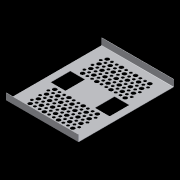
# Autodesk Inventor part: Belly Pan
Saved by Autodesk Inventor 2014 SP1 (Build 180222100, 222)
## iProperties
Created: 2013-11-29
Part Number: Belly Pan
Material: Aluminum 6061
Document SubType Name: Sheet Metal
Designer: Rauhul Varma
Mass: 3080.17 g
Surface Area: 7653.53 cm^2
Volume: 1136.59 cm^3
Density: 2.71 g/cm^3
Sheet Metal Rule: Default
Appearance: Aluminum - Flat
Flat Pattern Width: 55.88 cm
Flat Pattern Length: 83.9863 cm
Flat Pattern Area: 4693.16 cm^2
Sheet Metal Width: 22.000 in
Sheet Metal Length: 33.065 in
Sheet Metal Area: 727.441 in^2
Author: Rauhul Varma
Autodesk Inventor part; units mm, degrees
ref_plane "YZ Plane" through (0, 0, 0) normal (1, 0, 0) x (0, 1, 0)
ref_plane "XZ Plane" through (0, 0, 0) normal (0, 1, 0) x (-1, 0, 0)
sketch "Sketch2" plane through (0, 0, 0) normal (0, 1, 0) x (-1, 0, 0)
  line L0 (0, 0) -> (558.8, 0)
  line L1 (558.8, 0) -> (558.8, 736.6)
  line L2 (558.8, 736.6) -> (0, 736.6)
  line L3 (0, 736.6) -> (0, 0)
  line L4 (50.8, 736.6) -> (50.8, 0)
  line L5 (508, 736.6) -> (508, 0)
  line L6 (50.8, 698.5) -> (508, 698.5)
  line L7 (508, 38.1) -> (50.8, 38.1)
  line L8 (0, 368.3) -> (558.8, 368.3)
  line L9 (50.8, 444.5) -> (165.1, 444.5)
  line L10 (165.1, 444.5) -> (165.1, 292.1)
  line L11 (165.1, 292.1) -> (50.8, 292.1)
  line L12 (508, 292.1) -> (393.7, 292.1)
  line L13 (393.7, 292.1) -> (393.7, 444.5)
  line L14 (393.7, 444.5) -> (508, 444.5)
  line L15 (63.5, 698.5) -> (63.5, 457.2)
  line L16 (63.5, 457.2) -> (177.8, 457.2)
  line L17 (177.8, 457.2) -> (177.8, 279.4)
  line L18 (177.8, 279.4) -> (63.5, 279.4)
  line L19 (63.5, 279.4) -> (63.5, 38.1)
  line L20 (495.3, 698.5) -> (495.3, 457.2)
  line L21 (495.3, 457.2) -> (381, 457.2)
  line L22 (381, 457.2) -> (381, 279.4)
  line L23 (381, 279.4) -> (495.3, 279.4)
  line L24 (495.3, 279.4) -> (495.3, 38.1)
  circle A0 centre (85.725, 676.275) radius 22.225
  circle A1 centre (85.725, 598.805) radius 22.225
  circle A2 centre (85.725, 521.335) radius 22.225
  circle A3 centre (163.195, 676.275) radius 22.225
  circle A4 centre (163.195, 598.805) radius 22.225
  circle A5 centre (163.195, 521.335) radius 22.225
  circle A6 centre (240.665, 676.275) radius 22.225
  circle A7 centre (240.665, 598.805) radius 22.225
  circle A8 centre (240.665, 521.335) radius 22.225
  circle A9 centre (318.135, 676.275) radius 22.225
  circle A10 centre (318.135, 598.805) radius 22.225
  circle A11 centre (318.135, 521.335) radius 22.225
  circle A12 centre (395.605, 676.275) radius 22.225
  circle A13 centre (395.605, 598.805) radius 22.225
  circle A14 centre (395.605, 521.335) radius 22.225
  circle A15 centre (473.075, 676.275) radius 22.225
  circle A16 centre (473.075, 598.805) radius 22.225
  circle A17 centre (473.075, 521.335) radius 22.225
  circle A18 centre (85.725, 60.325) radius 22.225
  circle A19 centre (85.725, 137.795) radius 22.225
  circle A20 centre (85.725, 215.265) radius 22.225
  circle A21 centre (163.195, 60.325) radius 22.225
  circle A22 centre (163.195, 137.795) radius 22.225
  circle A23 centre (163.195, 215.265) radius 22.225
  circle A24 centre (240.665, 60.325) radius 22.225
  circle A25 centre (240.665, 137.795) radius 22.225
  circle A26 centre (240.665, 215.265) radius 22.225
  circle A27 centre (318.135, 60.325) radius 22.225
  circle A28 centre (318.135, 137.795) radius 22.225
  circle A29 centre (318.135, 215.265) radius 22.225
  circle A30 centre (395.605, 60.325) radius 22.225
  circle A31 centre (395.605, 137.795) radius 22.225
  circle A32 centre (395.605, 215.265) radius 22.225
  circle A33 centre (473.075, 60.325) radius 22.225
  circle A34 centre (473.075, 137.795) radius 22.225
  circle A35 centre (473.075, 215.265) radius 22.225
  line L25 (85.725, 676.275) -> (163.195, 598.805) construction
  line L26 (163.195, 676.275) -> (85.725, 598.805) construction
  circle A36 centre (124.46, 637.54) radius 17.4625
  circle A37 centre (124.46, 560.07) radius 17.4625
  circle A38 centre (201.93, 637.54) radius 17.4625
  circle A39 centre (201.93, 560.07) radius 17.4625
  circle A40 centre (279.4, 637.54) radius 17.4625
  circle A41 centre (279.4, 560.07) radius 17.4625
  circle A42 centre (356.87, 637.54) radius 17.4625
  circle A43 centre (356.87, 560.07) radius 17.4625
  circle A44 centre (434.34, 637.54) radius 17.4625
  circle A45 centre (434.34, 560.07) radius 17.4625
  line L27 (85.725, 60.325) -> (163.195, 137.795) construction
  line L28 (163.195, 60.325) -> (85.725, 137.795) construction
  circle A46 centre (124.46, 99.06) radius 17.4625
  circle A47 centre (124.46, 176.53) radius 17.4625
  circle A48 centre (201.93, 99.06) radius 17.4625
  circle A49 centre (201.93, 176.53) radius 17.4625
  circle A50 centre (279.4, 99.06) radius 17.4625
  circle A51 centre (279.4, 176.53) radius 17.4625
  circle A52 centre (356.87, 99.06) radius 17.4625
  circle A53 centre (356.87, 176.53) radius 17.4625
  circle A54 centre (434.34, 99.06) radius 17.4625
  circle A55 centre (434.34, 176.53) radius 17.4625
  dimension "d2" = 558.8
  dimension "d3" = 736.6
  dimension "d25" = 50.8
  dimension "d26" = 50.8
  dimension "d27" = 38.1
  dimension "d28" = 38.1
  dimension "d29" = 114.3
  dimension "d30" = 114.3
  dimension "d31" = 152.4
  dimension "d32" = 152.4
  dimension "d33" = 12.7
  dimension "d34" = 12.7
  dimension "d35" = 12.7
  dimension "d36" = 12.7
  dimension "d37" = 12.7
  dimension "d38" = 12.7
  dimension "d39" = 12.7
  dimension "d40" = 12.7
  dimension "d41" = 12.7
  dimension "d42" = 12.7
  dimension "d43" = 44.45
  dimension "d46" = 77.47
  dimension "d49" = 77.47
  dimension "d52" = 44.45
  dimension "d55" = 77.47
  dimension "d58" = 77.47
  dimension "d61" = 34.925
  dimension "d64" = 77.47
  dimension "d67" = 77.47
  dimension "d70" = 34.925
  dimension "d73" = 77.47
  dimension "d76" = 77.47
  constraints: 58 end point, 56 centre point, 16 point on line, 14 perpendicular, 8 parallel, 5 horizontal, 4 midpoint, 4 tangent, 4 vertical, 1 collinear, 106 other
  measures "d2" distance of L2.end L1.end
  measures "d3" distance of L1.end L0.end
  measures "d25" distance between parallel lines of L4 L3
  measures "d26" distance between parallel lines of L1 L5
  measures "d27" distance between parallel lines of L6 L2
  measures "d28" distance between parallel lines of L7 L0
  measures "d29" distance of L13.end L14.end
  measures "d30" distance of L9.start L9.end
  measures "d31" distance between parallel lines of L11 L9
  measures "d32" distance between parallel lines of L12 L14
  measures "d33" distance between parallel lines of L15 L4
  measures "d34" distance between parallel lines of L16 L9
  measures "d35" distance between parallel lines of L17 L10
  measures "d36" distance between parallel lines of L11 L18
  measures "d37" distance between parallel lines of L4 L19
  measures "d38" distance between parallel lines of L5 L20
  measures "d39" distance between parallel lines of L21 L14
  measures "d40" distance between parallel lines of L22 L13
  measures "d41" distance between parallel lines of L12 L23
  measures "d42" distance between parallel lines of L5 L24
  measures "d43" diameter of A0
  measures "d46" distance of L25.start L26.end
  measures "d49" distance of L25.start L26.start
  measures "d52" diameter of A18
  measures "d55" distance of L27.start L28.end
  measures "d58" distance of L27.start L28.start
  measures "d61" diameter of A36
  measures "d64" distance of A36.centre A37.centre
  measures "d67" distance of A36.centre A38.centre
  measures "d70" diameter of A46
  measures "d73" distance of A46.centre A47.centre
  measures "d76" distance of A46.centre A48.centre
extrude "Plate1" add sketch "Sketch2" along normal blind 3.175 contours L3 L8 L4 L0 | L4 L7 L5 L0 | L3 L2 L4 L8 | L5 L8 L1 L0 | L4 L11 L10 L8 L17 L18 L19 L7 | L8 L10 L11 L4 | L4 L9 L10 L8 | L7 L24 L23 L22 L8 L13 L12 L5 | L19 A18 L7 | L2 L5 L6 L4 | L4 L6 L15 L16 L17 L8 L10 L9 | L8 L5 L2 L1 | L12 L13 L8 L5 | L7 A33 L24 | A21 | A24 | A27 | A30 | A34 | A35 | A20 | A19 | A18 L19 L18 L17 L8 L22 L23 L24 A33 L7 | A18 | A17 | A16 | A12 | A9 | A6 | A3 | A1 | A2 | L17 L16 L15 A0 L6 A15 L20 L21 L22 L8 | L8 L13 L14 L5 | A33 | L5 L14 L13 L8 L22 L21 L20 L6 | L6 A0 L15 | L20 A15 L6 | A0 | A15 | A4 | A5 | A7 | A8 | A10 | A11 | A13 | A14 | A22 | A23 | A25 | A26 | A28 | A29 | A31 | A32 | A36 | A37 | A38 | A39 | A40 | A41 | A42 | A43 | A44 | A45 | A46 | A47 | A48 | A49 | A50 | A51 | A52 | A53 | A54 | A55
cut "Cut2" [suppressed]
sketch "Sketch12" plane through (0, 3.175, 736.6) normal (0, 0, 1) x (1, 0, 0)
  line L0 (-558.8, 0) -> (0, 0)
  line L1 (0, 0) -> (0, 50.8)
  line L2 (0, 50.8) -> (-558.8, 50.8)
  line L3 (-558.8, 50.8) -> (-558.8, 0)
  constraints: 6 end point, 1 horizontal, 1 perpendicular, 1 vertical
edge flange "Flange5" height 50.8 angle 90 thickness 3.175 bend radius 3.175 thickness toward (0, 0, 1) relief tear relief width 3.175 relief depth 1.5875 corner gap 3.175 corner form 0 edges at (-279.4, 3.175, 736.6) (-279.4, 3.175, 0) wall of the first edge with corners at (-558.8, 3.175, 736.6) (0, 3.175, 736.6) (0, 53.975, 736.6) (-558.8, 53.975, 736.6)
bend "Bend9"
corner "Corner5"
sketch "Sketch13" plane through (0, 3.175, 0) normal (0, 1, 0) x (1, 0, 0)
  line L0 (0, -3.175) -> (-558.8, -3.175) projected
  line L1 (-558.8, -733.425) -> (-558.8, -3.175) projected
  line L2 (-558.8, -733.425) -> (0, -733.425) projected
  line L3 (0, -3.175) -> (0, -733.425) projected
  line L4 (-165.1, -444.5) -> (-165.1, -292.1) projected
  line L5 (-165.1, -292.1) -> (-50.8, -292.1) projected
  line L6 (-50.8, -444.5) -> (-165.1, -444.5) projected
  line L7 (-50.8, -736.6) -> (-50.8, 0) projected
  line L8 (-508, -736.6) -> (-508, 0) projected
  line L9 (-393.7, -292.1) -> (-393.7, -444.5) projected
  line L10 (-508, -292.1) -> (-393.7, -292.1) projected
  line L11 (-393.7, -444.5) -> (-508, -444.5) projected
  line L12 (-558.8, -25.4) -> (0, -25.4)
  line L13 (-558.8, -711.2) -> (0, -711.2)
  line L14 (-50.8, -457.2) -> (-177.8, -457.2)
  line L15 (-177.8, -457.2) -> (-177.8, -279.4)
  line L16 (-177.8, -279.4) -> (-50.8, -279.4)
  line L17 (-508, -457.2) -> (-381, -457.2)
  line L18 (-381, -457.2) -> (-381, -279.4)
  line L19 (-381, -279.4) -> (-508, -279.4)
  line L20 (-558.8, -698.5) -> (0, -698.5)
  line L21 (-558.8, -38.1) -> (0, -38.1)
  line L22 (-481.0396, -279.4) -> (-481.0396, -38.1)
  line L23 (-77.7604, -279.4) -> (-77.7604, -38.1)
  line L24 (-77.7604, -457.2) -> (-77.7604, -698.5)
  line L25 (-481.0396, -457.2) -> (-481.0396, -698.5)
  line L26 (-426.047, -101.6) -> (-462.7087, -101.6) construction
  line L27 (-462.7087, -101.6) -> (-481.0396, -69.85) construction
  line L28 (-481.0396, -69.85) -> (-462.7087, -38.1) construction
  line L29 (-462.7087, -38.1) -> (-426.047, -38.1) construction
  line L30 (-426.047, -38.1) -> (-407.7161, -69.85) construction
  line L31 (-407.7161, -69.85) -> (-426.047, -101.6) construction
  circle A0 centre (-407.7161, -69.85) radius 11.1125
  circle A1 centre (-426.047, -101.6) radius 11.1125
  circle A2 centre (-462.7087, -101.6) radius 11.1125
  circle A3 centre (-444.3778, -69.85) radius 15.875
  circle A4 centre (-481.0396, -69.85) radius 11.1125 construction
  line L32 (-316.0617, -101.6) -> (-352.7235, -101.6) construction
  line L33 (-352.7235, -101.6) -> (-371.0544, -69.85) construction
  line L34 (-371.0544, -69.85) -> (-352.7235, -38.1) construction
  line L35 (-352.7235, -38.1) -> (-316.0617, -38.1) construction
  line L36 (-316.0617, -38.1) -> (-297.7309, -69.85) construction
  line L37 (-297.7309, -69.85) -> (-316.0617, -101.6) construction
  circle A5 centre (-297.7309, -69.85) radius 11.1125
  circle A6 centre (-316.0617, -101.6) radius 11.1125
  circle A7 centre (-352.7235, -101.6) radius 11.1125
  circle A8 centre (-334.3926, -69.85) radius 15.875
  circle A9 centre (-371.0544, -69.85) radius 11.1125
  line L38 (-206.0765, -101.6) -> (-242.7383, -101.6) construction
  line L39 (-242.7383, -101.6) -> (-261.0691, -69.85) construction
  line L40 (-261.0691, -69.85) -> (-242.7383, -38.1) construction
  line L41 (-242.7383, -38.1) -> (-206.0765, -38.1) construction
  line L42 (-206.0765, -38.1) -> (-187.7456, -69.85) construction
  line L43 (-187.7456, -69.85) -> (-206.0765, -101.6) construction
  circle A10 centre (-187.7456, -69.85) radius 11.1125
  circle A11 centre (-206.0765, -101.6) radius 11.1125
  circle A12 centre (-242.7383, -101.6) radius 11.1125
  circle A13 centre (-224.4074, -69.85) radius 15.875
  circle A14 centre (-261.0691, -69.85) radius 11.1125
  line L44 (-96.0913, -101.6) -> (-132.753, -101.6) construction
  line L45 (-132.753, -101.6) -> (-151.0839, -69.85) construction
  line L46 (-151.0839, -69.85) -> (-132.753, -38.1) construction
  line L47 (-132.753, -38.1) -> (-96.0913, -38.1) construction
  line L48 (-96.0913, -38.1) -> (-77.7604, -69.85) construction
  line L49 (-77.7604, -69.85) -> (-96.0913, -101.6) construction
  circle A15 centre (-77.7604, -69.85) radius 11.1125 construction
  circle A16 centre (-96.0913, -101.6) radius 11.1125
  circle A17 centre (-132.753, -101.6) radius 11.1125
  circle A18 centre (-114.4222, -69.85) radius 15.875
  circle A19 centre (-151.0839, -69.85) radius 11.1125
  line L50 (-426.047, -165.1) -> (-462.7087, -165.1) construction
  line L51 (-462.7087, -165.1) -> (-481.0396, -133.35) construction
  line L52 (-481.0396, -133.35) -> (-462.7087, -101.6) construction
  line L53 (-462.7087, -101.6) -> (-426.047, -101.6) construction
  line L54 (-426.047, -101.6) -> (-407.7161, -133.35) construction
  line L55 (-407.7161, -133.35) -> (-426.047, -165.1) construction
  circle A20 centre (-407.7161, -133.35) radius 11.1125
  circle A21 centre (-426.047, -165.1) radius 11.1125
  circle A22 centre (-462.7087, -165.1) radius 11.1125
  circle A23 centre (-444.3778, -133.35) radius 15.875
  circle A24 centre (-481.0396, -133.35) radius 11.1125 construction
  line L56 (-316.0617, -165.1) -> (-352.7235, -165.1) construction
  line L57 (-352.7235, -165.1) -> (-371.0544, -133.35) construction
  line L58 (-371.0544, -133.35) -> (-352.7235, -101.6) construction
  line L59 (-352.7235, -101.6) -> (-316.0617, -101.6) construction
  line L60 (-316.0617, -101.6) -> (-297.7309, -133.35) construction
  line L61 (-297.7309, -133.35) -> (-316.0617, -165.1) construction
  circle A25 centre (-297.7309, -133.35) radius 11.1125
  circle A26 centre (-316.0617, -165.1) radius 11.1125
  circle A27 centre (-352.7235, -165.1) radius 11.1125
  circle A28 centre (-334.3926, -133.35) radius 15.875
  circle A29 centre (-371.0544, -133.35) radius 11.1125
  line L62 (-206.0765, -165.1) -> (-242.7383, -165.1) construction
  line L63 (-242.7383, -165.1) -> (-261.0691, -133.35) construction
  line L64 (-261.0691, -133.35) -> (-242.7383, -101.6) construction
  line L65 (-242.7383, -101.6) -> (-206.0765, -101.6) construction
  line L66 (-206.0765, -101.6) -> (-187.7456, -133.35) construction
  line L67 (-187.7456, -133.35) -> (-206.0765, -165.1) construction
  circle A30 centre (-187.7456, -133.35) radius 11.1125
  circle A31 centre (-206.0765, -165.1) radius 11.1125
  circle A32 centre (-242.7383, -165.1) radius 11.1125
  circle A33 centre (-224.4074, -133.35) radius 15.875
  circle A34 centre (-261.0691, -133.35) radius 11.1125
  line L68 (-96.0913, -165.1) -> (-132.753, -165.1) construction
  line L69 (-132.753, -165.1) -> (-151.0839, -133.35) construction
  line L70 (-151.0839, -133.35) -> (-132.753, -101.6) construction
  line L71 (-132.753, -101.6) -> (-96.0913, -101.6) construction
  line L72 (-96.0913, -101.6) -> (-77.7604, -133.35) construction
  line L73 (-77.7604, -133.35) -> (-96.0913, -165.1) construction
  circle A35 centre (-77.7604, -133.35) radius 11.1125 construction
  circle A36 centre (-96.0913, -165.1) radius 11.1125
  circle A37 centre (-132.753, -165.1) radius 11.1125
  circle A38 centre (-114.4222, -133.35) radius 15.875
  circle A39 centre (-151.0839, -133.35) radius 11.1125
  line L74 (-426.047, -228.6) -> (-462.7087, -228.6) construction
  line L75 (-462.7087, -228.6) -> (-481.0396, -196.85) construction
  line L76 (-481.0396, -196.85) -> (-462.7087, -165.1) construction
  line L77 (-462.7087, -165.1) -> (-426.047, -165.1) construction
  line L78 (-426.047, -165.1) -> (-407.7161, -196.85) construction
  line L79 (-407.7161, -196.85) -> (-426.047, -228.6) construction
  circle A40 centre (-407.7161, -196.85) radius 11.1125
  circle A41 centre (-426.047, -228.6) radius 11.1125
  circle A42 centre (-462.7087, -228.6) radius 11.1125
  circle A43 centre (-444.3778, -196.85) radius 15.875
  circle A44 centre (-481.0396, -196.85) radius 11.1125 construction
  line L80 (-316.0617, -228.6) -> (-352.7235, -228.6) construction
  line L81 (-352.7235, -228.6) -> (-371.0544, -196.85) construction
  line L82 (-371.0544, -196.85) -> (-352.7235, -165.1) construction
  line L83 (-352.7235, -165.1) -> (-316.0617, -165.1) construction
  line L84 (-316.0617, -165.1) -> (-297.7309, -196.85) construction
  line L85 (-297.7309, -196.85) -> (-316.0617, -228.6) construction
  circle A45 centre (-297.7309, -196.85) radius 11.1125
  circle A46 centre (-316.0617, -228.6) radius 11.1125
  circle A47 centre (-352.7235, -228.6) radius 11.1125
  circle A48 centre (-334.3926, -196.85) radius 15.875
  circle A49 centre (-371.0544, -196.85) radius 11.1125
  line L86 (-206.0765, -228.6) -> (-242.7383, -228.6) construction
  line L87 (-242.7383, -228.6) -> (-261.0691, -196.85) construction
  line L88 (-261.0691, -196.85) -> (-242.7383, -165.1) construction
  line L89 (-242.7383, -165.1) -> (-206.0765, -165.1) construction
  line L90 (-206.0765, -165.1) -> (-187.7456, -196.85) construction
  line L91 (-187.7456, -196.85) -> (-206.0765, -228.6) construction
  circle A50 centre (-187.7456, -196.85) radius 11.1125
  circle A51 centre (-206.0765, -228.6) radius 11.1125
  circle A52 centre (-242.7383, -228.6) radius 11.1125
  circle A53 centre (-224.4074, -196.85) radius 15.875
  circle A54 centre (-261.0691, -196.85) radius 11.1125
  line L92 (-96.0913, -228.6) -> (-132.753, -228.6) construction
  line L93 (-132.753, -228.6) -> (-151.0839, -196.85) construction
  line L94 (-151.0839, -196.85) -> (-132.753, -165.1) construction
  line L95 (-132.753, -165.1) -> (-96.0913, -165.1) construction
  line L96 (-96.0913, -165.1) -> (-77.7604, -196.85) construction
  line L97 (-77.7604, -196.85) -> (-96.0913, -228.6) construction
  circle A55 centre (-77.7604, -196.85) radius 11.1125 construction
  circle A56 centre (-96.0913, -228.6) radius 11.1125
  circle A57 centre (-132.753, -228.6) radius 11.1125
  circle A58 centre (-114.4222, -196.85) radius 15.875
  circle A59 centre (-151.0839, -196.85) radius 11.1125
  line L98 (-426.047, -292.1) -> (-462.7087, -292.1) construction
  line L99 (-462.7087, -292.1) -> (-481.0396, -260.35) construction
  line L100 (-481.0396, -260.35) -> (-462.7087, -228.6) construction
  line L101 (-462.7087, -228.6) -> (-426.047, -228.6) construction
  line L102 (-426.047, -228.6) -> (-407.7161, -260.35) construction
  line L103 (-407.7161, -260.35) -> (-426.047, -292.1) construction
  circle A60 centre (-407.7161, -260.35) radius 11.1125
  circle A61 centre (-426.047, -292.1) radius 11.1125 construction
  circle A62 centre (-462.7087, -292.1) radius 11.1125 construction
  circle A63 centre (-444.3778, -260.35) radius 15.875
  circle A64 centre (-481.0396, -260.35) radius 11.1125 construction
  line L104 (-316.0617, -292.1) -> (-352.7235, -292.1) construction
  line L105 (-352.7235, -292.1) -> (-371.0544, -260.35) construction
  line L106 (-371.0544, -260.35) -> (-352.7235, -228.6) construction
  line L107 (-352.7235, -228.6) -> (-316.0617, -228.6) construction
  line L108 (-316.0617, -228.6) -> (-297.7309, -260.35) construction
  line L109 (-297.7309, -260.35) -> (-316.0617, -292.1) construction
  circle A65 centre (-297.7309, -260.35) radius 11.1125
  circle A66 centre (-316.0617, -292.1) radius 11.1125 construction
  circle A67 centre (-352.7235, -292.1) radius 11.1125 construction
  circle A68 centre (-334.3926, -260.35) radius 15.875
  circle A69 centre (-371.0544, -260.35) radius 11.1125
  line L110 (-206.0765, -292.1) -> (-242.7383, -292.1) construction
  line L111 (-242.7383, -292.1) -> (-261.0691, -260.35) construction
  line L112 (-261.0691, -260.35) -> (-242.7383, -228.6) construction
  line L113 (-242.7383, -228.6) -> (-206.0765, -228.6) construction
  line L114 (-206.0765, -228.6) -> (-187.7456, -260.35) construction
  line L115 (-187.7456, -260.35) -> (-206.0765, -292.1) construction
  circle A70 centre (-187.7456, -260.35) radius 11.1125
  circle A71 centre (-206.0765, -292.1) radius 11.1125 construction
  circle A72 centre (-242.7383, -292.1) radius 11.1125 construction
  circle A73 centre (-224.4074, -260.35) radius 15.875
  circle A74 centre (-261.0691, -260.35) radius 11.1125
  line L116 (-96.0913, -292.1) -> (-132.753, -292.1) construction
  line L117 (-132.753, -292.1) -> (-151.0839, -260.35) construction
  line L118 (-151.0839, -260.35) -> (-132.753, -228.6) construction
  line L119 (-132.753, -228.6) -> (-96.0913, -228.6) construction
  line L120 (-96.0913, -228.6) -> (-77.7604, -260.35) construction
  line L121 (-77.7604, -260.35) -> (-96.0913, -292.1) construction
  circle A75 centre (-77.7604, -260.35) radius 11.1125 construction
  circle A76 centre (-96.0913, -292.1) radius 11.1125 construction
  circle A77 centre (-132.753, -292.1) radius 11.1125 construction
  circle A78 centre (-114.4222, -260.35) radius 15.875
  circle A79 centre (-151.0839, -260.35) radius 11.1125
  line L122 (-407.7161, -133.35) -> (-371.0544, -69.85) construction
  circle A80 centre (-389.3852, -101.6) radius 15.875
  circle A81 centre (-279.4, -101.6) radius 15.875
  circle A82 centre (-169.4148, -101.6) radius 15.875
  circle A83 centre (-389.3852, -165.1) radius 15.875
  circle A84 centre (-279.4, -165.1) radius 15.875
  circle A85 centre (-169.4148, -165.1) radius 15.875
  circle A86 centre (-389.3852, -228.6) radius 15.875
  circle A87 centre (-279.4, -228.6) radius 15.875
  circle A88 centre (-169.4148, -228.6) radius 15.875
  point P0 (0, 0)
  dimension "d156" = 22.225
  dimension "d157" = 22.225
  dimension "d158" = 12.7
  dimension "d159" = 12.7
  dimension "d160" = 12.7
  dimension "d161" = 12.7
  dimension "d162" = 26.9604
  dimension "d163" = 26.9604
  dimension "d164" = 26.9604
  dimension "d165" = 26.9604
  dimension "d166" = 63.5
  dimension "d167" = 403.2792
  dimension "d169" = 22.225
  dimension "d170" = 22.225
  dimension "d171" = 22.225
  dimension "d173" = 31.75
  dimension "d174" = 22.225
  dimension "d179" = 109.9852
  dimension "d182" = 63.5
  dimension "d186" = 31.75
  dimension "d189" = 109.9852
  dimension "d192" = 63.5
  constraints: 222 end point, 89 centre point, 65 coincident, 14 point on line, 5 perpendicular, 3 horizontal, 3 parallel, 2 vertical, 1 midpoint, 363 other
  measures "d156" distance between parallel lines of L0 L12
  measures "d157" distance between parallel lines of L13 L2
  measures "d158" distance between parallel lines of L12 L21
  measures "d159" distance between parallel lines of L20 L13
  measures "d160" distance between parallel lines of L11 L17
  measures "d161" distance between parallel lines of L6 L14
  measures "d162" distance between parallel lines of L8 L25
  measures "d163" distance between parallel lines of L7 L24
  measures "d164" distance between parallel lines of L7 L23
  measures "d165" distance between parallel lines of L8 L22
  measures "d166" distance between parallel lines of L29 L26
  measures "d167" distance between parallel lines of L23 L22
  measures "d169" diameter of A0
  measures "d170" diameter of A1
  measures "d171" diameter of A2
  measures "d173" diameter of A3
  measures "d174" diameter of A4
  measures "d179" distance of L27.end L34.start
  measures "d182" distance of L27.end L52.start
  measures "d186" diameter of A80
  measures "d189" distance of A80.centre A81.centre
  measures "d192" distance of A80.centre A83.centre
extrude "Cheese Holes" cut sketch "Sketch13" against normal blind 3.175 contours A0 | A1 | A2 | A3 | A5 | A6 | A7 | A8 | A9 | A10 | A11 | A12 | A13 | A14 | A16 | A17 | A18 | A19 | A20 | A21 | A22 | A23 | A25 | A26 | A27 | A28 | A29 | A30 | A31 | A32 | A33 | A34 | A36 | A37 | A38 | A39 | A40 | A41 | A42 | A43 | A45 | A46 | A47 | A48 | A49 | A50 | A51 | A52 | A53 | A54 | A56 | A57 | A58 | A59 | A60 | A63 | A65 | A68 | A69 | A70 | A73 | A74 | A78 | A79 | A80 | A81 | A82 | A83 | A84 | A85 | A86 | A87 | A88
extrude "Gearboxes Cutouts" cut sketch "Sketch13" against normal blind 3.175 contours L7 L6 L4 L5 | L10 L9 L11 L8
ref_plane "MidPlane" through (-558.8, 53.975, 368.3) normal (0, 0, 1) x (1, 0, 0)
mirror "Mirror1" about plane through (-558.8, 53.975, 368.3) normal (0, 0, 1) of "Cheese Holes"
equation "\"d46\" = d49"
equation "\"d55\" = d46"
equation "\"d58\" = d55"
equation "\"d64\" = d46"
equation "\"d67\" = d49"
equation "\"d73\" = d55"
equation "\"d76\" = d58"
equation "\"d83\" = Thickness"
equation "\"d162\" = d165"
equation "\"d163\" = d165"
equation "\"d164\" = d165"
equation "\"d169\" = d174"
equation "\"d170\" = d174"
equation "\"d171\" = d174"
equation "\"d186\" = d173"
equation "\"d195\" = Thickness"
equation "\"d197\" = Thickness"
equation "\"d146\" = BendReliefWidth"
equation "\"d147\" = BendReliefDepth"
equation "\"d148\" = MinimumRemnant"
equation "\"d149\" = BendRadius"
equation "\"d152\" = BendRadius"
equation "\"d153\" = CornerReliefSize"
equation "\"d154\" = GapSize"
equation "\"d155\" = JacobiRadiusSize"
equation "\"BendRadius\" = Thickness"
equation "\"BendReliefWidth\" = Thickness"
equation "\"BendReliefDepth\" = 0.5 * Thickness"
equation "\"CornerReliefSize\" = 4 * Thickness"
equation "\"MinimumRemnant\" = 2 * Thickness"
equation "\"TransitionRadius\" = BendRadius"
equation "\"JacobiRadiusSize\" = BendRadius"
equation "\"GapSize\" = Thickness"
equation "\"d4\" = BendRadius"
equation "\"root2\" = 1.414214"
equation "\"Thickness\" = 3.175"
body "Solid1"
